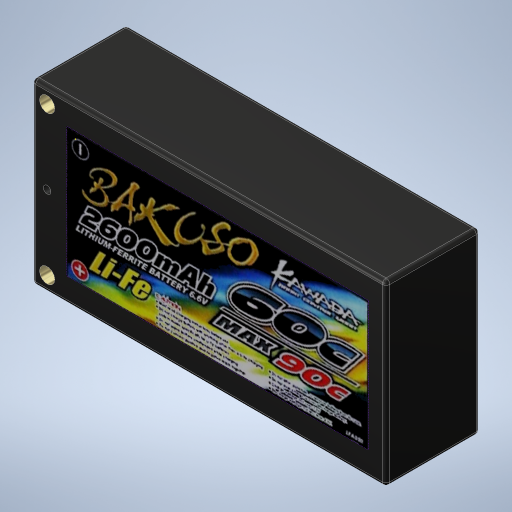
# Autodesk Inventor part: バッテリー BAKUSO
Saved by Autodesk Inventor 2023.1 (Build 271208000, 208)
## iProperties
Created: 2018-09-30
Part Number: バッテリー BAKUSO
Material: 一般
Document SubType Name: Modeling
Designer: tanjihayato
Density: 1.63077 g/cm^3
Appearance: 光沢 - 黒
Mass: 175 g
Surface Area: 156.649 cm^2
Volume: 107.311 cm^3
Author: tanjihayato
Autodesk Inventor part; units mm, degrees
ref_plane "YZ Plane" through (0, 0, 0) normal (1, 0, 0) x (0, 1, 0)
ref_plane "XZ Plane" through (0, 0, 0) normal (0, 1, 0) x (-1, 0, 0)
ref_plane "XY Plane" through (0, 0, 0) normal (0, 0, 1) x (1, 0, 0)
sketch "スケッチ1" plane through (0, 0, 0) normal (0, 0, 1) x (1, 0, 0)
  line L0 (-11.4461, 8.1838) -> (81.5539, 8.1838)
  line L1 (81.5539, 8.1838) -> (81.5539, -38.7162)
  line L2 (81.5539, -38.7162) -> (-11.4461, -38.7162)
  line L3 (-11.4461, -38.7162) -> (-11.4461, 8.1838)
  point P0 (0, 0)
  dimension "d0" = 93
  dimension "d1" = 46.9
  constraints: 8 end point, 2 parallel, 1 horizontal, 1 perpendicular
  measures "d0" distance of L1.end L2.end
  measures "d1" distance of L0.end L1.end
extrude "押し出し1" add sketch "スケッチ1" along normal blind 24.7
fillet "フィレット1" radius 1 12 edges at (35.0539, 8.1838, 24.7) (-11.4461, -15.2662, 24.7) (-11.4461, 8.1838, 12.35) (35.0539, -38.7162, 24.7) (-11.4461, -38.7162, 12.35) (35.0539, -38.7162, 0) (81.5539, -38.7162, 12.35) (81.5539, -15.2662, 24.7) (81.5539, 8.1838, 12.35) (81.5539, -15.2662, 0) (35.0539, 8.1838, 0) (-11.4461, -15.2662, 0)
sketch "スケッチ2" plane through (0, 0, 24.7) normal (0, 0, 1) x (1, 0, 0)
  line L0 (-10.4461, -37.7162) -> (-10.4461, 7.1838) projected
  line L1 (80.5539, -37.7162) -> (-10.4461, -37.7162) projected
  line L2 (80.5539, 7.1838) -> (80.5539, -37.7162) projected
  line L3 (-10.4461, 7.1838) -> (80.5539, 7.1838) projected
  circle A0 centre (-7.4461, 4.1838) radius 2
  circle A1 centre (-7.4461, -34.7162) radius 2
  line L4 (-0.4461, 2.1838) -> (75.5539, 2.1838)
  line L5 (75.5539, 2.1838) -> (75.5539, -32.7162)
  line L6 (75.5539, -32.7162) -> (-0.4461, -32.7162)
  line L7 (-0.4461, -32.7162) -> (-0.4461, 2.1838)
  circle A2 centre (-7.4461, -15.2662) radius 1
  point P0 (0, 0)
  dimension "d5" = 4
  dimension "d6" = 4
  dimension "d7" = 3
  dimension "d8" = 3
  dimension "d9" = 3
  dimension "d10" = 3
  dimension "d11" = 5
  dimension "d12" = 5
  dimension "d13" = 5
  dimension "d14" = 10
  dimension "d15" = 2
  constraints: 8 end point, 3 centre point, 2 parallel, 1 horizontal, 1 perpendicular
  measures "d5" diameter of A0
  measures "d6" diameter of A1
  measures "d7" distance from line of L1 A1.centre
  measures "d8" distance from line of L0 A1.centre
  measures "d9" distance from line of L3 A0.centre
  measures "d10" distance from line of L0 A0.centre
  measures "d11" distance between parallel lines of L4 L3
  measures "d12" distance between parallel lines of L1 L6
  measures "d13" distance between parallel lines of L2 L5
  measures "d14" distance between parallel lines of L7 L0
  measures "d15" diameter of A2
extrude "押し出し2" cut sketch "スケッチ2" against normal blind 10 contours A0 | A1 | A2
sketch "スケッチ3" plane through (0, 0, 24.7) normal (0, 0, 1) x (1, 0, 0)
  line L0 (-2.3175, 1.7393) -> (76.8469, 1.7393) construction
  line L1 (76.8469, 1.7393) -> (76.8469, -32.2836) construction
  line L2 (76.8469, -32.2836) -> (-2.3175, -32.2836) construction
  line L3 (-2.3175, -32.2836) -> (-2.3175, 1.7393) construction
  point P0 (0, 0)
  constraints: 2 other
